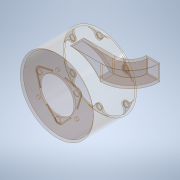
# Autodesk Inventor part: Dust Bin
Saved by Autodesk Inventor 2020 (Build 240168000, 168)
## iProperties
Created: 2020-03-28
Part Number: Dust Bin
Material: Generic
Document SubType Name: Modeling
Designer: pengpeng
Density: 1 g/cm^3
Appearance: Polycarbonate - Smoked
Author: pengpeng
Autodesk Inventor part; units mm, degrees
ref_plane "YZ Plane" through (0, 0, 0) normal (1, 0, 0) x (0, 1, 0)
ref_plane "XY Plane" through (0, 0, 0) normal (0, 0, 1) x (1, 0, 0)
sketch "Sketch1" plane through (0, 0, 0) normal (0, 0, 1) x (1, 0, 0)
  circle A0 centre (0, 0) radius 68
  dimension "d1" = 136
  constraints: 1 centre point
  measures "d1" diameter of A0
extrude "Extrusion1" add sketch "Sketch1" along normal blind 80
shell "Shell1" thickness 3 removed faces 1 at (13.6377, 7.7647, 0)
sketch "Sketch2" plane through (0, 0, 80) normal (0, 0, 1) x (1, 0, 0)
  circle A0 centre (0, 0) radius 32
  dimension "d5" = 64
  constraints: 1 centre point, 1 coincident
  measures "d5" diameter of A0
extrude "Extrusion2" cut sketch "Sketch2" against normal up to surface (3 mm away)
sketch "Sketch3" plane through (0, 0, 77) normal (0, 0, -1) x (-1, 0, 0)
  circle A0 centre (0, 0) radius 32 projected
  circle A1 centre (0, 0) radius 65 projected
  circle A2 centre (0, -40) radius 4.8
  line L0 (0, 0) -> (0, -56.282) construction
  line L1 (0, 0) -> (-47.9956, 27.7103) construction
  line L2 (0, 0) -> (60.1339, 34.7183) construction
  circle A3 centre (-34.641, 20) radius 4.8
  circle A4 centre (34.641, 20) radius 4.8
  dimension "d8" = 9.6
  dimension "d9" = 40
  dimension "d10" = 120
  dimension "d11" = 120
  dimension "d12" = 9.6
  dimension "d13" = 9.6
  dimension "d14" = 40
  dimension "d15" = 40
  constraints: 6 end point, 3 centre point, 2 point on line, 1 vertical
  measures "d8" diameter of A2
  measures "d9" distance of point (0, 0) A2.centre
  measures "d10" angle of L0 L1
  measures "d11" angle of L0 L2
  measures "d12" diameter of A3
  measures "d13" diameter of A4
  measures "d14" distance of point (0, 0) A4.centre
  measures "d15" distance of point (0, 0) A3.centre
extrude "Extrusion3" cut sketch "Sketch3" against normal blind 1.524 contours A2 | A3 | A4
ref_plane "Work Plane1" through (0, 0, 55) normal (0, 0, 1) x (1, 0, 0)
sketch "Sketch4" plane through (0, 0, 55) normal (0, 0, 1) x (1, 0, 0)
  circle A0 centre (0, 0) radius 68 projected
  circle A1 centre (0, 0) radius 68 projected
  line L0 (0, 68) -> (56.3915, 68)
  line L1 (56.3915, 68) -> (56.3915, 38)
  line L2 (56.3915, 38) -> (0, 38)
  line L3 (0, 38) -> (0, 68)
  dimension "d24" = 30
  constraints: 8 end point, 2 horizontal, 2 parallel, 1 perpendicular, 1 vertical alignment, 3 other
  measures "d24" distance between parallel lines of L2 L0
extrude "Extrusion4" add sketch "Sketch4" against normal blind 25 contours A0 L0 L1
sketch "Sketch6" plane through (56.3915, 38, 55) normal (1, 0, 0) x (0, 0, -1)
  line L0 (0, 0) -> (0, 30) projected
  line L1 (25, 0) -> (0, 0) projected
  line L2 (25, 30) -> (25, 0) projected
  line L3 (0, 30) -> (25, 30) projected
  line L4 (22, 27) -> (22, 3)
  line L5 (22, 3) -> (3, 3)
  line L6 (3, 3) -> (3, 27)
  line L7 (3, 27) -> (22, 27)
  point P0 (55, -38)
  dimension "d27" = 3
  constraints: 8 end point, 3 other
  measures "d27" distance between parallel lines of L3 L7
extrude "Extrusion5" cut sketch "Sketch6" against normal blind 56.391 contours L4 L5 L6 L7
ref_plane "Work Plane4" through (0, 68, 0) normal (0, 1, 0) x (-1, 0, 0)
sketch "Sketch9" plane through (56.3915, 38, 55) normal (1, 0, 0) x (0, 0, -1)
  line L0 (3, 3) -> (3, 27) projected
  line L1 (3, 27) -> (22, 27) projected
  line L2 (22, 27) -> (22, 3) projected
  line L3 (22, 3) -> (3, 3) projected
  line L4 (0, 0) -> (0, 30) projected
  line L5 (25, 0) -> (0, 0) projected
  line L6 (25, 30) -> (25, 0) projected
  line L7 (0, 30) -> (25, 30) projected
  point P0 (55, -38)
sketch "Sketch10" plane through (0, 68, 0) normal (0, 1, 0) x (-1, 0, 0)
  circle A0 centre (-56.3915, 0) radius 55 construction
  line L0 (-127.7058, 55) -> (100.6176, 55) projected
  line L1 (-56.3915, 55) -> (0, 55) projected
  line L2 (0, 0) -> (-96.3915, 0) construction
  arc A1 (-56.3915, 55) -> (-111.3915, 0) centre (-56.3915, 0) ccw
  constraints: 4 point on circle, 2 centre point, 2 coincident, 2 end point, 1 horizontal, 1 point on line, 1 tangent
sweep "Sweep2" add profiles "Sketch9" path "Sketch10" path curves A1
sketch "Sketch11" plane through (0, 0, 77) normal (0, 0, -1) x (-1, 0, 0)
  circle A0 centre (-34.641, 20) radius 4.8 projected
  circle A1 centre (34.641, 20) radius 4.8 projected
  circle A2 centre (0, -40) radius 4.8 projected
  circle A3 centre (0, 0) radius 32 projected
  circle A4 centre (0, 0) radius 65 projected
  circle A5 centre (-34.641, 20) radius 6.3
  circle A6 centre (34.641, 20) radius 6.3
  circle A7 centre (0, -40) radius 6.3
  circle A8 centre (0, 0) radius 33.5
  line L0 (-36.0415, 26.1424) -> (-7.4468, 32.6618)
  line L1 (-40.6607, 18.1416) -> (-32.0094, -9.8818)
  line L2 (36.0415, 26.1424) -> (7.4468, 32.6618)
  line L3 (40.6607, 18.1416) -> (32.0094, -9.8818)
  line L4 (4.6192, -44.284) -> (24.5626, -22.78)
  line L5 (-4.6192, -44.284) -> (-24.5626, -22.78)
  circle A9 centre (-34.641, 20) radius 7.8
  line L6 (-42.0939, 17.6992) -> (-34.7194, -6.1884)
  circle A10 centre (34.641, 20) radius 7.8
  circle A11 centre (0, -40) radius 7.8
  line L7 (-36.3749, 27.6048) -> (-12.0004, 33.1621)
  line L8 (36.3749, 27.6048) -> (12.0004, 33.1621)
  line L9 (42.0939, 17.6992) -> (34.7194, -6.1884)
  line L10 (5.7191, -45.304) -> (22.7191, -26.9737)
  line L11 (-5.7191, -45.304) -> (-22.7191, -26.9737)
  line L12 (-34.7194, -6.1884) -> (-33.2862, -5.746)
  line L13 (-22.7191, -26.9737) -> (-21.6192, -25.9537)
  line L14 (12.0004, 33.1621) -> (11.6669, 31.6997)
  line L15 (34.7194, -6.1884) -> (33.2862, -5.746)
  line L16 (22.7191, -26.9737) -> (21.6192, -25.9537)
  line L17 (-12.0004, 33.1621) -> (-11.6669, 31.6997)
  dimension "d94" = 360
  dimension "d39" = 1.5
  dimension "d40" = 1.5
  dimension "d41" = 1.5
  dimension "d42" = 1.5
  dimension "d43" = 1.5
  dimension "d44" = 1.5
  dimension "d45" = 1.5
  dimension "d46" = 25
  dimension "d47" = 25
  dimension "d48" = 25
  dimension "d49" = 25
  dimension "d50" = 25
  dimension "d51" = 25
  constraints: 36 end point, 18 point on circle, 18 tangent, 7 centre point, 6 parallel, 6 perpendicular, 6 point on line
  measures "d39" radial gap between concentric circles of A0 A5
  measures "d40" radial gap between concentric circles of A1 A6
  measures "d41" radial gap between concentric circles of A2 A7
  measures "d42" radial gap between concentric circles of A8 A3
  measures "d43" radial gap between concentric circles of A5 A9
  measures "d44" radial gap between concentric circles of A6 A10
  measures "d45" radial gap between concentric circles of A7 A11
  measures "d46" distance of L6.start L6.end
  measures "d47" distance of L7.start L7.end
  measures "d48" distance of L8.start L8.end
  measures "d49" distance of L9.start L9.end
  measures "d50" distance of L10.start L10.end
  measures "d51" distance of L11.start L11.end
extrude "Extrusion6" add sketch "Sketch11" along normal blind 1.5 contours A5 L1 A9 L0 | A9 L7 L17 L0 | L1 L12 L6 A9 | L14 L8 A10 L2 | L5 A11 L11 L13 | A10 L3 A6 L2 | L5 A7 L4 A11 | A10 L9 L15 L3 | L16 L10 A11 L4
sketch "Sketch12" plane through (0, 0, 0) normal (0, 0, -1) x (-1, 0, 0)
  circle A0 centre (0, 0) radius 65 projected
  circle A1 centre (0, 0) radius 68 projected
  line L0 (0, 0) -> (0, 89.9409) construction
  line L1 (0, 0) -> (-80.2223, -46.3164) construction
  line L2 (0, 0) -> (82.1519, -47.4304) construction
  line L3 (0, 0) -> (99.5929, 57.5) construction
  line L4 (0, 0) -> (-70.8187, 40.8872) construction
  line L5 (-70.8187, 40.8872) -> (0, 0) construction
  line L6 (0, 0) -> (0, -89.6127) construction
  circle A2 centre (0, 57.5) radius 4.8
  circle A3 centre (49.7965, 28.75) radius 4.8
  circle A4 centre (49.7965, -28.75) radius 4.8
  circle A5 centre (0, -57.5) radius 4.8
  circle A6 centre (-49.7965, -28.75) radius 4.8
  circle A7 centre (-49.7965, 28.75) radius 4.8
  circle A8 centre (-49.7965, 28.75) radius 6.3
  circle A9 centre (0, 57.5) radius 6.3
  circle A10 centre (49.7965, 28.75) radius 6.3
  circle A11 centre (49.7965, -28.75) radius 6.3
  circle A12 centre (0, -57.5) radius 6.3
  circle A13 centre (-49.7965, -28.75) radius 6.3
  circle A14 centre (-37.8823, 39.874) radius 10
  circle A15 centre (-53.473, 12.87) radius 10
  circle A16 centre (-15.5907, 52.744) radius 10
  circle A17 centre (15.5907, 52.744) radius 10
  circle A18 centre (37.8823, 39.874) radius 10
  circle A19 centre (53.473, 12.87) radius 10
  circle A20 centre (53.473, -12.87) radius 10
  circle A21 centre (37.8823, -39.874) radius 10
  circle A22 centre (15.5907, -52.744) radius 10
  circle A23 centre (-15.5907, -52.744) radius 10
  circle A24 centre (-37.8823, -39.874) radius 10
  circle A25 centre (-53.473, -12.87) radius 10
  circle A26 centre (0, 0) radius 65 projected
  point P0 (-6.0259, -55.6618)
  point P1 (-18.4254, -62.3338)
  point P2 (18.4254, -62.3338)
  point P3 (6.0259, -55.6618)
  point P4 (45.1916, -33.0494)
  point P5 (44.77, -47.1238)
  point P6 (63.1954, -15.2101)
  point P7 (51.2175, -22.6123)
  point P8 (51.2175, 22.6123)
  point P9 (63.1954, 15.2101)
  point P10 (44.77, 47.1238)
  point P11 (45.1916, 33.0494)
  point P12 (6.0259, 55.6618)
  point P13 (18.4254, 62.3338)
  point P14 (-18.4254, 62.3338)
  point P15 (-6.0259, 55.6618)
  point P16 (-63.1954, 15.2101)
  point P17 (-51.2175, 22.6123)
  point P18 (-45.1916, 33.0494)
  point P19 (-44.77, 47.1238)
  point P20 (-51.2175, -22.6123)
  point P21 (-63.1954, -15.2101)
  point P22 (-44.77, -47.1238)
  point P23 (-45.1916, -33.0494)
  dimension "d54" = 120
  dimension "d55" = 120
  dimension "d56" = 120
  dimension "d57" = 120
  dimension "d58" = 9.6
  dimension "d59" = 9.6
  dimension "d60" = 9.6
  dimension "d61" = 9.6
  dimension "d62" = 9.6
  dimension "d63" = 9.6
  dimension "d64" = 57.5
  dimension "d65" = 57.5
  dimension "d66" = 57.5
  dimension "d67" = 57.5
  dimension "d68" = 57.5
  dimension "d69" = 57.5
  dimension "d70" = 1.5
  dimension "d71" = 1.5
  dimension "d72" = 1.5
  dimension "d73" = 1.5
  dimension "d74" = 1.5
  dimension "d75" = 1.5
  dimension "d76" = 20
  dimension "d77" = 20
  dimension "d78" = 20
  dimension "d79" = 20
  dimension "d80" = 20
  dimension "d81" = 20
  dimension "d82" = 20
  dimension "d83" = 20
  dimension "d84" = 20
  dimension "d85" = 20
  dimension "d86" = 20
  dimension "d87" = 20
  constraints: 24 centre point, 24 tangent, 14 end point, 5 point on line, 2 vertical, 1 collinear, 1 midpoint
  measures "d54" angle of L0 L1
  measures "d55" angle of L2 L1
  measures "d56" angle of L6 L3
  measures "d57" angle of L4 L3
  measures "d58" diameter of A2
  measures "d59" diameter of A7
  measures "d60" diameter of A6
  measures "d61" diameter of A5
  measures "d62" diameter of A4
  measures "d63" diameter of A3
  measures "d64" distance of point (0, 0) A2.centre
  measures "d65" distance of point (0, 0) A3.centre
  measures "d66" distance of point (0, 0) A4.centre
  measures "d67" distance of point (0, 0) A5.centre
  measures "d68" distance of A0.centre A6.centre
  measures "d69" distance of A7.centre point (0, 0)
  measures "d70" radial gap between concentric circles of A8 A7
  measures "d71" radial gap between concentric circles of A2 A9
  measures "d72" radial gap between concentric circles of A3 A10
  measures "d73" radial gap between concentric circles of A4 A11
  measures "d74" radial gap between concentric circles of A5 A12
  measures "d75" radial gap between concentric circles of A6 A13
  measures "d76" diameter of A14
  measures "d77" diameter of A15
  measures "d78" diameter of A16
  measures "d79" diameter of A17
  measures "d80" diameter of A18
  measures "d81" diameter of A19
  measures "d82" diameter of A20
  measures "d83" diameter of A21
  measures "d84" diameter of A22
  measures "d85" diameter of A23
  measures "d86" diameter of A24
  measures "d87" diameter of A25
extrude "Extrusion7" add sketch "Sketch12" against normal blind 3 contours A19 A10 A18 A0 | A0 A21 A11 A20 | A10 | A11 | A17 A9 A16 A0 | A0 A23 A12 A22 | A9 | A12 | A14 A8 A15 A0 | A0 A25 A13 A24 | A8 | A13 | A1 | A2 | A3 | A4 | A5 | A6 | A7
sketch "Sketch13" plane through (0, 0, 0) normal (0, 0, -1) x (-1, 0, 0)
  circle A0 centre (0, 0) radius 68 projected
  line L0 (0, 0) -> (0, 119.968) construction
  circle A1 centre (0, 57.5) radius 4.8
  line L1 (0, 0) -> (-103.8953, 59.984) construction
  circle A2 centre (-49.7965, 28.75) radius 4.8
  line L2 (0, 0) -> (-103.8953, -59.984) construction
  circle A3 centre (-49.7965, -28.75) radius 4.8
  line L3 (0, 0) -> (0, -119.968) construction
  circle A4 centre (0, -57.5) radius 4.8
  line L4 (0, 0) -> (103.8953, -59.984) construction
  circle A5 centre (49.7965, -28.75) radius 4.8
  line L5 (0, 0) -> (103.8953, 59.984) construction
  circle A6 centre (49.7965, 28.75) radius 4.8
  dimension "d90" = 9.6
  dimension "d91" = 57.5
  dimension "d94" = 360
  constraints: 12 end point, 6 centre point, 6 point on line, 1 vertical, 31 other
  measures "d90" diameter of A1
  measures "d91" distance of point (0, 0) A1.centre
extrude "Extrusion8" cut sketch "Sketch13" against normal blind 1.524 contours A1 | A2 | A3 | A4 | A5 | A6
sketch "Sketch14" plane through (0, 0, 80) normal (0, 0, 1) x (1, 0, 0)
  circle A0 centre (0, 0) radius 32 projected
  line L0 (0, 0) -> (0, 28.9416) construction
  circle A1 centre (0, 41) radius 3
  line L1 (0, 0) -> (-25.0642, -14.4708) construction
  line L2 (0, 0) -> (25.0642, -14.4708) construction
  point P0 (-35.507, -20.5)
  point P1 (-35.507, -20.5)
  point P2 (35.507, -20.5)
  point P3 (35.507, -20.5)
  dimension "d98" = 6
  dimension "d99" = 41
  dimension "d102" = 360
  constraints: 6 end point, 3 coincident, 3 point on line, 1 centre point, 1 vertical, 16 other
  measures "d98" diameter of A1
  measures "d99" distance of point (0, 0) A1.centre
hole "Hole1" at (0, 41, 80) at (-35.507, -20.5, 80) at (35.507, -20.5, 80) direction (0, 0, -1) diameter 6 end through all
equation "\"d11\" = d10"
equation "\"d12\" = d8"
equation "\"d13\" = d8"
equation "\"d14\" = d9"
equation "\"d15\" = d9"
equation "\"d40\" = d39"
equation "\"d41\" = d39"
equation "\"d42\" = d39"
equation "\"d44\" = d43"
equation "\"d45\" = d41"
equation "\"d47\" = d46"
equation "\"d48\" = d47"
equation "\"d49\" = d48"
equation "\"d50\" = d49"
equation "\"d51\" = d50"
equation "\"d55\" = d54"
equation "\"d56\" = d54"
equation "\"d57\" = d54"
equation "\"d59\" = d58"
equation "\"d60\" = d58"
equation "\"d61\" = d58"
equation "\"d62\" = d58"
equation "\"d63\" = d58"
equation "\"d65\" = d64"
equation "\"d66\" = d64"
equation "\"d67\" = d64"
equation "\"d68\" = d64"
equation "\"d69\" = d64"
equation "\"d71\" = d70"
equation "\"d72\" = d70"
equation "\"d73\" = d70"
equation "\"d74\" = d70"
equation "\"d75\" = d70"
equation "\"d77\" = d76"
equation "\"d78\" = d76"
equation "\"d79\" = d76"
equation "\"d80\" = d76"
equation "\"d81\" = d76"
equation "\"d82\" = d76"
equation "\"d83\" = d76"
equation "\"d84\" = d83"
equation "\"d85\" = d76"
equation "\"d86\" = d76"
equation "\"d87\" = d76"
body "Solid1"
